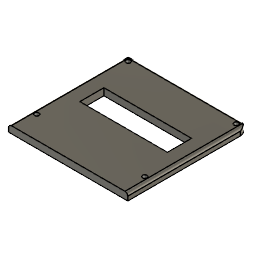
Wake Up Top (Autodesk Fusion 360 design; units mm, degrees)
part number: 2026-08-26-20-39-43-190
Autodesk Fusion 360 part; units mm, degrees
note: some values were not read from the file. Set by a fixed rule: which face or edge a step refers to.
sketch "Sketch1" plane through (0, 0, 0) normal (0, 0, 1) x (1, 0, 0)
  line L0 (0, 0) -> (84.406, 0)
  line L1 (84.406, 0) -> (84.406, 84.71)
  line L2 (84.406, 84.71) -> (0, 84.71)
  line L3 (0, 84.71) -> (0, 0)
  dimension "d1" = 84.406
  dimension "d2" = 84.71
  constraint horizontal L0
  constraint vertical L1
  constraint horizontal L2
  constraint vertical L3
  constraint coincident L0.start L3.end
  measures "d1" distance of L0.start L0.end
  measures "d2" distance of L0.start L2.end
sketch "Sketch2" plane through (0, 0, 0) normal (0, 0, 1) x (1, 0, 0)
  line L0 (0, 0) -> (84.406, 0)
  line L1 (84.406, 0) -> (84.406, 84.71)
  line L2 (84.406, 84.71) -> (0, 84.71)
  line L3 (0, 84.71) -> (0, 0)
  dimension "d11" = 84.406
  dimension "d12" = 84.71
  constraint horizontal L0
  constraint vertical L1
  constraint horizontal L2
  constraint vertical L3
  constraint coincident L0.start L3.end
  measures "d11" distance of L0.start L0.end
  measures "d12" distance of L0.start L2.end
extrude "Extrude2" add sketch "Sketch2" along normal blind 5
sketch "Sketch3" plane through (0, 0, 5) normal (0, 0, 1) x (-1, 0, 0)
  line L0 (0, -84.71) -> (0, 0)
  line L1 (0, 0) -> (-84.406, 0)
  line L2 (-84.406, 0) -> (-84.406, -84.71)
  line L3 (-84.406, -84.71) -> (0, -84.71)
  circle A0 centre (-4, -80.71) radius 1.6
  circle A1 centre (-80.406, -80.71) radius 1.6
  circle A2 centre (-80.406, -16) radius 1.6
  circle A3 centre (-4, -16) radius 1.6
  dimension "d15" = 3.2
  dimension "d16" = 3.2
  dimension "d17" = 3.2
  dimension "d18" = 3.2
  dimension "d19" = 4
  dimension "d20" = 4
  dimension "d21" = 4
  dimension "d22" = 4
  dimension "d23" = 4
  dimension "d24" = 4
  dimension "d25" = 16
  dimension "d26" = 16
  measures "d15" diameter of A0
  measures "d16" diameter of A1
  measures "d17" diameter of A2
  measures "d18" diameter of A3
  measures "d19" distance of L3 A0.centre
  measures "d20" distance of L0 A0.centre
  measures "d21" distance of L2 A1.centre
  measures "d22" distance of L3 A1.centre
  measures "d23" distance of L0 A3.centre
  measures "d24" distance of L2 A2.centre
  measures "d25" distance of L1 A2.centre
  measures "d26" distance of L1 A3.centre
extrude "Extrude3" cut sketch "Sketch3" against normal blind 110 contours A0 | A1 | A2 | A3
fillet "Fillet4" radius 5 1 edges at (84.406, 84.71, 2.5)
fillet "Fillet5" radius 5 1 edges at (0, 84.71, 2.5)
fillet "Fillet6" radius 2 5 edges at (84.406, 39.855, 5) (82.9415, 83.2455, 5) (42.203, 84.71, 5) (1.4645, 83.2455, 5) (0, 39.855, 5)
delete_face "DeleteFace1" 3 faces at (4.7744, 84.6687, 3.3785) (1.7275, 82.9825, 4.1618) (0.0545, 79.935, 3.4417)
delete_face "DeleteFace2" 3 faces at (79.631, 84.6555, 3.4417) (82.6785, 82.9825, 4.1618) (84.3647, 79.9356, 3.3785)
sketch "Sketch4" plane through (0, 0, 5) normal (0, 0, 1) x (-1, 0, 0)
  circle A0 centre (-80.406, -80.71) radius 1.6
  circle A1 centre (-4, -16) radius 1.6
  circle A2 centre (-4, -80.71) radius 1.6
  circle A3 centre (-80.406, -16) radius 1.6
  line L0 (-82.406, -82.71) -> (-2, -82.71)
  line L1 (-2, -82.71) -> (-2, 0)
  line L2 (-2, 0) -> (-82.406, 0)
  line L3 (-82.406, 0) -> (-82.406, -82.71)
  line L4 (-11.5, -56) -> (-73.5, -56)
  line L5 (-73.5, -56) -> (-73.5, -40)
  line L6 (-73.5, -40) -> (-11.5, -40)
  line L7 (-11.5, -40) -> (-11.5, -56)
  dimension "d35" = 62
  dimension "d36" = 16
  dimension "d37" = 40
  dimension "d38" = 9.5
  constraint horizontal L4
  constraint vertical L5
  constraint horizontal L6
  constraint vertical L7
  measures "d35" distance of L4.start L4.end
  measures "d36" distance of L4.start L6.end
  measures "d37" distance of L2 L6
  measures "d38" distance of L1 L7
extrude "Extrude4" cut sketch "Sketch4" against normal blind 15 contours L4 L5 L6 L7
sketch "Sketch5" plane through (0, 0, 5) normal (0, 0, 1) x (-1, 0, 0)
  line L0 (-73.5, -56) -> (-73.5, -40)
  line L1 (-73.5, -40) -> (-11.5, -40)
  line L2 (-11.5, -40) -> (-11.5, -56)
  line L3 (-11.5, -56) -> (-73.5, -56)
  circle A0 centre (-80.406, -80.71) radius 1.6
  circle A1 centre (-4, -16) radius 1.6
  circle A2 centre (-4, -80.71) radius 1.6
  circle A3 centre (-80.406, -16) radius 1.6
  line L4 (-82.406, -82.71) -> (-2, -82.71)
  line L5 (-2, -82.71) -> (-2, 0)
  line L6 (-2, 0) -> (-82.406, 0)
  line L7 (-82.406, 0) -> (-82.406, -82.71)
  line L8 (-11.5, -40) -> (-73.5, -40)
  line L9 (-73.5, -40) -> (-73.5, -39)
  line L10 (-73.5, -39) -> (-11.5, -39)
  line L11 (-11.5, -39) -> (-11.5, -40)
  dimension "d41" = 1
  constraint horizontal L8
  constraint vertical L9
  constraint horizontal L10
  constraint vertical L11
  constraint coincident L1.end L2.start
  measures "d41" distance of L1.end L10.end
extrude "Extrude5" cut sketch "Sketch5" against normal blind 40 contours L1 L8 L9 L10 L11
